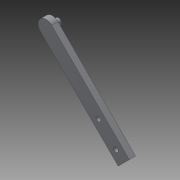
# Autodesk Inventor part: eye_tracker_angled_arm
Saved by Autodesk Inventor 2015 (Build 190159000, 159)
## iProperties
Created: 2015-06-20
Part Number: eye_tracker_angled_arm
Material: Generic
Document SubType Name: Modeling
Designer: Master
Density: 1 g/cm^3
Appearance: Default
Author: Master
Autodesk Inventor part; units mm, degrees
ref_plane "YZ Plane" through (0, 0, 0) normal (1, 0, 0) x (0, 1, 0)
ref_plane "XZ Plane" through (0, 0, 0) normal (0, 1, 0) x (-1, 0, 0)
ref_plane "XY Plane" through (0, 0, 0) normal (0, 0, 1) x (1, 0, 0)
sketch "Sketch1" plane through (0, 0, 0) normal (0, 0, 1) x (1, 0, 0)
  circle A0 centre (1.9895, 47.0752) radius 2 projected
  line L0 (-3.9007, 3) -> (-3.9007, 30) projected
  line L1 (-3.9007, 40) -> (-3.9007, 55) projected
  circle A1 centre (1.9895, 47.0752) radius 5
  line L2 (1.9895, 47.0752) -> (-1.546, 43.5397)
  line L3 (1.9895, 47.0752) -> (6.9895, 47.0752) construction
  line L4 (1.9895, 47.0752) -> (5.525, 50.6108)
  arc A2 (1.9895, 1.5) -> (47.0122, 40) centre (1.9895, 47.0752) ccw projected
  arc A3 (1.9895, -1.5) -> (50.0467, 40) centre (1.9895, 47.0752) ccw projected
  line L5 (-1.546, 43.5397) -> (47.9514, -5.9578)
  line L6 (5.525, 50.6108) -> (55.0225, 1.1133)
  line L7 (47.9514, -5.9578) -> (55.0225, 1.1133)
  circle A4 centre (35.2767, 13.788) radius 1.5
  point P0 (0, 0)
  dimension "d0" = 10
  dimension "d1" = 135
  dimension "d3" = 10
  dimension "d4" = 3
  dimension "d5" = 5
  dimension "d6" = 70
  constraints: 12 end point, 2 centre point, 2 parallel, 2 point on circle, 1 coincident, 1 equal length, 1 horizontal, 1 perpendicular, 1 tangent
  measures "d0" diameter of A1
  measures "d1" angle of L2 L3
  measures "d3" distance between parallel lines of L5 L6
  measures "d4" diameter of A4
  measures "d5" distance from line of A4.centre L6
  measures "d6" distance between parallel lines of L4 L7
extrude "Extrusion1" add sketch "Sketch1" along normal blind 4 contours A0 L2 L4 | A0 L4 A1 L2 | L4 L2 A0 | A0 L2 A1 L4 | L6 A2 L5 A1 | L6 A3 A4 A2 | A2 A4 A3 L5 | L6 L7 L5 A3
sketch "Sketch2" plane through (0, 0, 0) normal (0, 0, -1) x (-1, 0, 0)
  circle A0 centre (-1.9895, 47.0752) radius 2 projected
  circle A1 centre (-1.9895, 47.0752) radius 1.85
  point P0 (0, 0)
  dimension "d9" = 3.7
  constraints: 1 centre point, 1 coincident
  measures "d9" diameter of A1
extrude "Extrusion2" add sketch "Sketch2" along normal blind 4 contours A1
sketch "Sketch3" plane through (0, 0, 4) normal (0, 0, 1) x (1, 0, 0)
  circle A0 centre (35.2767, 13.788) radius 1.5 projected
  arc A1 (5.525, 50.6108) -> (-1.546, 43.5397) centre (1.9895, 47.0752) ccw projected
  line L0 (-1.546, 43.5397) -> (47.9514, -5.9578) projected
  line L1 (47.9514, -5.9578) -> (55.0225, 1.1133) projected
  line L2 (55.0225, 1.1133) -> (5.525, 50.6108) projected
  circle A2 centre (46.5372, 2.5275) radius 1.5
  line L3 (35.2767, 13.788) -> (51.487, -2.4222)
  line L4 (47.9514, -5.9578) -> (55.0225, 1.1133) projected
  line L5 (55.0225, 1.1133) -> (5.525, 50.6108) projected
  point P0 (0, 0)
  dimension "d12" = 3
  dimension "d13" = 7
  constraints: 2 end point, 1 centre point, 1 midpoint, 1 parallel, 1 point on line
  measures "d12" diameter of A2
  measures "d13" distance from line of A2.centre L1
extrude "Extrusion3" cut sketch "Sketch3" against normal through all contours A2 L3 | L3 A2
body "Solid1"
